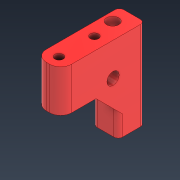
# Autodesk Inventor part: CH_01_0040_kradex_mount_2
Saved by Autodesk Inventor 2022.3 (Build 263350030, 350C)
## iProperties
Created: 2022-05-25
Part Number: CH_01_0040_kradex_mount_2
Material: Generic
Document SubType Name: Modeling
Designer: Tomasz Krakowski
Density: 1 g/cm^3
Appearance: Light Red
Author: Tomasz Krakowski
Autodesk Inventor part; units mm, degrees
ref_plane "YZ Plane" through (0, 0, 0) normal (1, 0, 0) x (0, 1, 0)
ref_plane "XZ Plane" through (0, 0, 0) normal (0, 1, 0) x (-1, 0, 0)
ref_plane "XY Plane" through (0, 0, 0) normal (0, 0, 1) x (1, 0, 0)
sketch "Sketch1" plane through (0, 0, 0) normal (0, 1, 0) x (-1, 0, 0)
  line L0 (-5.75, 13.75) -> (5.75, 13.75)
  line L1 (5.75, 13.75) -> (5.75, -13.75)
  line L2 (5.75, -13.75) -> (-5.75, -13.75)
  line L3 (-5.75, -13.75) -> (-5.75, 13.75)
  line L4 (-5.75, 13.75) -> (5.75, -13.75) construction
  line L5 (5.75, 13.75) -> (-5.75, -13.75) construction
  line L6 (0, 8) -> (0, -8) construction
  point P0 (0, 0)
  point P1 (0, 0)
  dimension "d0" = 16
  dimension "d18" = 27.5
  dimension "d19" = 11.5
  constraints: 14 end point, 8 point on line, 4 midpoint, 2 parallel, 1 horizontal, 1 perpendicular, 1 vertical
  measures "d0" distance of L6.start L6.end
  measures "d18" distance of L0.end L1.end
  measures "d19" distance between parallel lines of L3 L1
extrude "Extrusion1" add sketch "Sketch1" along normal blind 19
fillet "Fillet1" radius 5 2 edges at (5.75, 9.5, 13.75) (-5.75, 9.5, 13.75)
sketch "Sketch3" plane through (0, 19, 0) normal (0, 1, 0) x (1, 0, 0)
  line L0 (0, 7.25) -> (0, -8.75) construction
  line L1 (-5.75, 13.75) -> (-5.75, -8.75) construction
  line L2 (-0.75, -13.75) -> (0.75, -13.75) projected
  point P0 (0, 0)
  dimension "d7" = 16
  dimension "d8" = 5.75
  dimension "d9" = 5
  constraints: 2 end point, 1 vertical
  measures "d7" distance of L0.end L0.start
  measures "d8" distance between parallel lines of L0 L1
  measures "d9" distance from line of L2 L0.end
hole "Hole1" at (0, 19, -7.25) at (0, 19, 8.75) direction (0, -1, 0) diameter 3.8 depth 8
sketch "Sketch4" plane through (-5.75, 0, -13.75) normal (-1, 0, 0) x (0, 0, 1)
  line L0 (27.5, 0) -> (27.5, 19) projected
  point P0 (13.75, 0)
  point P1 (3.85, 4.1)
  dimension "d17" = 23.65
  dimension "d20" = 4.1
  measures "d17" distance from line of L0 point (3.85, 4.1)
  measures "d20" vertical distance of point (13.75, 0) point (3.85, 4.1)
hole "Hole2" at (-5.75, 4.1, -9.9) direction (1, 0, 0) diameter 5.5 end through all
sketch "Sketch5" plane through (0, 19, 0) normal (0, 1, 0) x (1, 0, 0)
  line L0 (5.75, 13.75) -> (-5.75, 13.75) construction
  line L1 (-5.75, 13.75) -> (5.75, 13.75)
  line L2 (5.75, 13.75) -> (5.75, 24.25)
  line L3 (5.75, 24.25) -> (-5.75, 24.25)
  line L4 (-5.75, 24.25) -> (-5.75, 13.75)
  line L5 (-0.75, -13.75) -> (0.75, -13.75) projected
  point P0 (0, 0)
  point P1 (0, -13.75)
  dimension "d28" = 38
  constraints: 8 end point, 2 parallel, 1 horizontal, 1 midpoint, 1 perpendicular
  measures "d28" distance from line of L3 point (0, -13.75)
extrude "Extrusion2" add sketch "Sketch5" against normal up to surface (19 mm away)
sketch "Sketch7" plane through (0, 19, 0) normal (0, 1, 0) x (1, 0, 0)
  circle A0 centre (0, 7.25) radius 1.9 construction
  circle A1 centre (0, -8.75) radius 1.9 construction
  point P0 (0, 0)
  point P1 (-1.75, 17.25)
  dimension "d31" = 1.75
  dimension "d32" = 10
  measures "d31" horizontal distance of point (-1.75, 17.25) A0.centre
  measures "d32" vertical distance of point (-1.75, 17.25) A0.centre
hole "Hole3" at (-1.75, 19, -17.25) direction (0, -1, 0) diameter 5.5 depth 8
sketch "Sketch9" plane through (0, 0, 0) normal (0, -1, 0) x (1, 0, 0)
  line L0 (5.75, 8.75) -> (5.75, -24.25) construction
  line L1 (-5.75, -24.25) -> (-5.75, 8.75) construction
  line L2 (5.75, -24.25) -> (-5.75, -24.25)
  line L3 (-5.75, -24.25) -> (-5.75, -12.25)
  line L4 (-5.75, -12.25) -> (5.75, -12.25)
  line L5 (5.75, -12.25) -> (5.75, -24.25)
  point P0 (0, 0)
  dimension "d47" = 12
  constraints: 8 end point, 2 parallel, 1 horizontal, 1 perpendicular, 1 point on line
  measures "d47" distance between parallel lines of L2 L4
extrude "Extrusion3" add sketch "Sketch9" along normal blind 21
chamfer "Chamfer1" distance 10 angle 45 1 edges at (0, 0, -12.25)
sketch "Sketch10" plane through (0, -21, 0) normal (0, -1, 0) x (1, 0, 0)
  circle A0 centre (-1.75, -17.25) radius 2.75 construction
  point P0 (0, 0)
  constraints: 1 coincident
hole "Hole5" at (-1.75, -21, -17.25) direction (0, 1, 0) diameter 5.5 depth 8
fillet "Fillet2" radius 2 4 edges at (-5.75, -1, -24.25) (5.75, -1, -24.25) (-5.75, -15.5, -12.25) (5.75, -15.5, -12.25)
body "Solid1"
